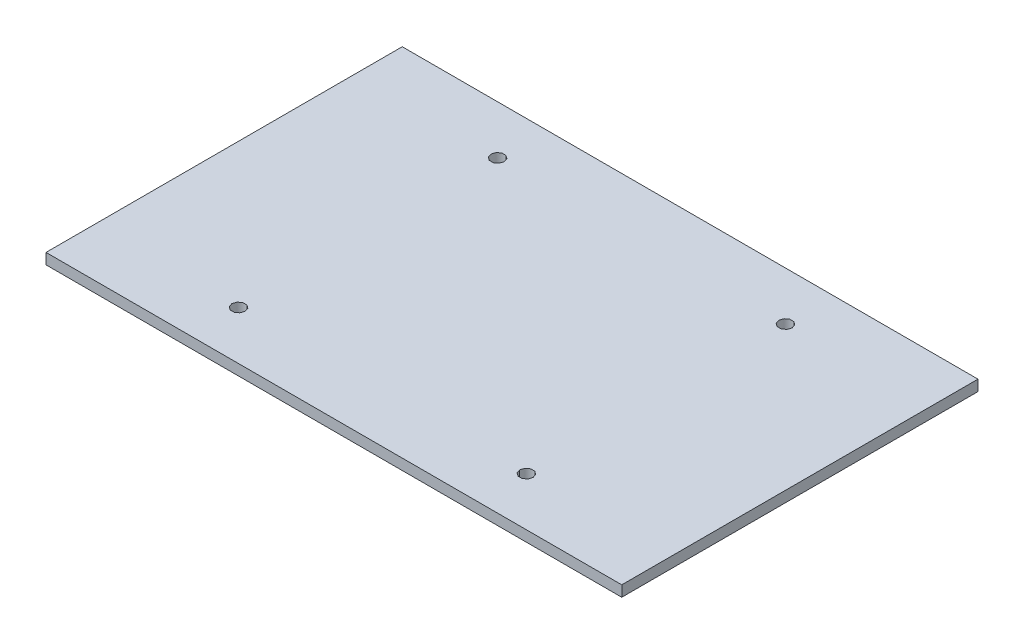
# Autodesk Inventor part: KB33-046-004-001 - Центральная пластина
Saved by Autodesk Inventor 2020 (Build 240168000, 168)
## iProperties
Created: 2021-06-25
Part Number: KB33-046-004-001 - Центральная пластина
Material: Типовые
Document SubType Name: Modeling
Designer: Петров Иван
Mass: 47.391 g
Surface Area: 332.875 cm^2
Volume: 47.391 cm^3
Density: 1 g/cm^3
Appearance: По умолчанию
Author: Петров Иван
Autodesk Inventor part; units mm, degrees
ref_plane "YZ Plane" through (0, 0, 0) normal (1, 0, 0) x (0, 1, 0)
ref_plane "XZ Plane" through (0, 0, 0) normal (0, 1, 0) x (-1, 0, 0)
ref_plane "XY Plane" through (0, 0, 0) normal (0, 0, 1) x (1, 0, 0)
sketch "Эскиз1" plane through (0, 0, 0) normal (0, 1, 0) x (-1, 0, 0)
  circle A0 centre (-40, 85.5) radius 1.85
  circle A1 centre (-40, 13.5) radius 1.85
  circle A2 centre (-120, 85.5) radius 1.85
  circle A3 centre (-120, 13.5) radius 1.85
  line L0 (0, 99) -> (0, 68.3189)
  line L1 (0, 99) -> (-160, 99)
  line L2 (-160, 0) -> (0, 0)
  line L3 (-160, 30.6811) -> (-160, 0)
  line L4 (0, 99) -> (-160, 99)
  line L5 (-160, 99) -> (-160, 0)
  line L6 (-160, 0) -> (0, 0)
  line L7 (0, 0) -> (0, 99)
  constraints: 16 end point, 4 centre point, 2 parallel, 1 horizontal, 1 perpendicular
extrude "Выдавливание1" add sketch "Эскиз1" along normal blind 3
